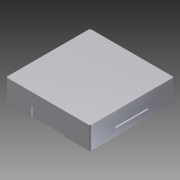
# Autodesk Inventor part: YB16SKW01-05-BB-BBni_lens
Saved by Autodesk Inventor 2014 (Build 180170000, 170)
## iProperties
Category: PARTsolutions
Company: NKKSWITCHES
Created: 2013-12-31
Part Number: YB16SKW01-05-BB-BBni_lens
Catalog Web Link: www.cadenas.de
Description: Panel Mount Non-Illuminated Pushbuttons_ni_lens-
Vendor: NKKSWITCHES
Document SubType Name: Modeling
Designer: PARTuser1
Manufacturer: NKKSWITCHES
Density: 1 g/cm^3
Material: Generic
Appearance: RGB(255.00000000000000,255.00000000000000,255.00000000000000)
PSOL_IDENT_0: {$CADENAS_DATA\23d-libs\nkkswitches\pushbuttons\yb\parts\yb_ni_lens.prj},283 {VTYP=3D},{NB=YB16SKW01
PSOL_IDENT_1: -05-BB-BBni_lens},{LINA=YB16SKW01-05-BB-BBni_lens},{NN=Panel Mount Non-Illuminated Pushbuttons_ni_le
PSOL_IDENT_2: ns},{DATE=23.07.2008 06:28:57},{GEOMDATE=23.07.2008 06:28:00},{VERSION=},{LINEID=10},{LINESUBID=-1},
PSOL_IDENT_3: {WBVAR=PLS,CRCTS,PS,SHPS,CMR,TRMNLS,LMPS,RSSTR,CTCLR,CCLR}  {NB=YB16SKW01-05-BB-BBni_lens},{LINA=YB1
PSOL_IDENT_4: 6SKW01-05-BB-BBni_lens},{KT=DUMMY},{PN=YB16SKW01-05-BB-BB},{SRS=YB},{PLS=1},{CRCTS=6},{PS=},{SHPS=S}
PSOL_IDENT_5: ,{SHPSALG= 'S', 'S - Square (Bushing Mounting)', 'C'  , 'C - Round (Bushing Mounting)', 'R', 'R - Re
PSOL_IDENT_6: ctangular (Bushing Mounting)'  , 'K', 'K - Square (Snap-in Mounting)', 'M', 'M - Round (Snap-in Moun
PSOL_IDENT_7: ting)'  , 'N', 'N - Rectangular (Snap-in Mounting)' },{HSNG=K - Black only},{CMR=W},{TRMNLS=01},{A=0
PSOL_IDENT_8: .709},{A1=0.591},{A11=0.827},{B=0.709},{B1=0.591},{L=0.669},{L1=0.327},{L2=0.957},{L3=0.429},{L4=0.3
PSOL_IDENT_9: 70},{L5=0.118},{L6=0.209},{L7=0.157},{L8=0.480},{DIA1=0.591},{DIA=0.709},{LMPS=05},{LMPS1= '05','05
PSOL_IDENT_10: - 5-volt (Incandescent Lamp used with Solid Cap)', '12','12 - 12-volt (Incandescent Lamp used with S
PSOL_IDENT_11: olid Cap)', '01','01 - 110-volt (Neon used w/ Insert Cap)', '05','05 - 5-volt (Incandescent used w/
PSOL_IDENT_12: Insert Cap)', '12','12 - 12-volt (Incandescent used w/ Insert Cap)', '5C','5C - Red (Bright LED used
PSOL_IDENT_13: with LED Cap)', '5D','5D - Amber (Bright LED used with LED Cap)', '5F','5F - Green (Bright LED used
PSOL_IDENT_14: with LED Cap)', '6B','6B - White (Super Bright LED used with LED Cap)', '6F','6F - Green (Super Bri
PSOL_IDENT_15: ght LED used with LED Cap)', '6G','6G - Blue (Super Bright LED used with LED Cap)', '1C','1C - Red S
PSOL_IDENT_16: ingle Color (LED in Spot Illuminated Cap)', '1D','1D - Amber Single Color (LED in Spot Illuminated C
PSOL_IDENT_17: ap)', '1F','1F - Green Single Color (LED in Spot Illuminated Cap)', 'CF','CF - Red/Green Bicolor (LE
PSOL_IDENT_18: D in Spot Illuminated Cap)' },{RSSTR=},{RSSTR1= '','N/A' },{CTCLR=BB},{CTCLR1= 'BB','BB - White/Whit
PSOL_IDENT_19: e (Solid Cap: Lens/Insert Colors)', 'CB','CB - Red/White (Solid Cap: Lens/Insert Colors)', 'EB','EB
PSOL_IDENT_20: - Yellow/White (Solid Cap: Lens/Insert Colors)', 'FB','FB - Green/White (Solid Cap: Lens/Insert Colo
PSOL_IDENT_21: rs)', 'GB','GB - Blue/White (Solid Cap: Lens/Insert Colors)' },{COLTRANS=1.00,1.00,1.00,0.00},{OCHR=
PSOL_IDENT_22: Download pdf},{NDM=16.000},{COL=1.00,1.00,1.00,0.00},{CCLR=BB}
CNS_NN: Panel Mount Non-Illuminated Pushbuttons_ni_lens
CNS_NB: YB16SKW01-05-BB-BBni_lens
CNS_NBSYN: $PN.ni_lens
CNS_LINA: YB16SKW01-05-BB-BBni_lens
CNS_PN: YB16SKW01-05-BB-BB
CNS_SRS: YB
CNS_PLS: 1 - SPDT
CNS_CRCTS: 6 - ON/ON
CNS_PS: Without Panel Seal
CNS_SHPS: S - Square (Bushing Mounting)
CNS_SHPSALG: 'S', 'S - Square (Bushing Mounting)', 'C'  , 'C - Round (Bushing Mounting)', 'R', 'R - Rectangular (Bushing Mounting)'  , 'K', 'K - Square (Snap-in Mounting)', 'M', 'M - Round (Snap-in Mounting)'  , 'N', 'N - Rectangular (Snap-in Mounting)'
CNS_HSNG: K - Black only
CNS_CMR: W - Silver; Rated 3A @ 125V AC
CNS_TRMNLS: 01 - Solder Lug/.110" (2.8mm) Quick Connect
CNS_A: 0.709
CNS_A1: 0.591
CNS_A11: 0.827
CNS_B: 0.709
CNS_B1: 0.591
CNS_L: 0.669
CNS_L1: 0.327
CNS_L2: 0.957
CNS_L3: 0.429
CNS_L4: 0.370
CNS_L5: 0.118
CNS_L6: 0.209
CNS_L7: 0.157
CNS_L8: 0.480
CNS_DIA1: 0.591
CNS_DIA: 0.709
CNS_LMPS: 05 - 5-volt (Incandescent Lamp for Solid Cap)
CNS_LMPS1: '05','05 - 5-volt (Incandescent Lamp used with Solid Cap)', '12','12 - 12-volt (Incandescent Lamp used with Solid Cap)', '01','01 - 110-volt (Neon used w/ Insert Cap)', '05','05 - 5-volt (Incandescent used w/ Insert Cap)', '12','12 - 12-volt (Incandescent used w/ Insert Cap)', '5C','5C - Red (Bright LED used with LED Cap)', '5D','5D - Amber (Bright LED used with LED Cap)', '5F','5F - Green (Bright LED used with LED Cap)', '6B','6B - White (Super Bright LED used with LED Cap)', '6F','6F - Green (Super Bright LED used with LED Cap)', '6G','6G - Blue (Super Bright LED used with LED Cap)', '1C','1C - Red Single Color (LED in Spot Illuminated Cap)', '1D','1D - Amber Single Color (LED in Spot Illuminated Cap)', '1F','1F - Green Single Color (LED in Spot Illuminated Cap)', 'CF','CF - Red/Green Bicolor (LED in Spot Illuminated Cap)'
CNS_RSSTR: N/A
CNS_RSSTR1: '','N/A'
CNS_CTCLR: BB - White/White (Solid Cap: Lens/Insert Colors)
CNS_CTCLR1: 'BB','BB - White/White (Solid Cap: Lens/Insert Colors)', 'CB','CB - Red/White (Solid Cap: Lens/Insert Colors)', 'EB','EB - Yellow/White (Solid Cap: Lens/Insert Colors)', 'FB','FB - Green/White (Solid Cap: Lens/Insert Colors)', 'GB','GB - Blue/White (Solid Cap: Lens/Insert Colors)'
CNS_COLTRANS: 1.00,1.00,1.00,0.00
CNS_OCHR: Download pdf
CNS_NDM: 16.000
CNS_COL: 1.00,1.00,1.00,0.00
CNS_CCLR: BB - White/White
SUPPLIER: NKKSWITCHES
ARTICLENO: YB16SKW01-05-BB-BBni_lens
BOMINFO: YB16SKW01-05-BB-BBni_lens
CREATOR: CADENAS GmbH
Title: YB16SKW01-05-BB-BBni_lens
Author: Cadenas PARTsolutions
Autodesk Inventor part; units mm, degrees
sketch "Sketch_31" plane through (0, 0, 0) normal (0, 0, 1) x (1, 0, 0)
  line L0 (-7.5057, 3.9878) -> (-7.5057, 0)
  line L1 (-7.5057, 0) -> (7.5057, 0)
  line L2 (7.5057, 0) -> (7.5057, 3.9878)
  line L3 (7.5057, 3.9878) -> (-7.5057, 3.9878)
  constraints: 8 end point
extrude "Extrusion1" add sketch "Sketch_31" along normal mid plane 15.0114
sketch "Sketch_4" plane through (0, 0, 0) normal (0, 0, 1) x (1, 0, 0)
  line L0 (-7.5057, 1.27) -> (-7.2517, 1.27)
  line L1 (-7.2517, 1.27) -> (-7.2517, 1.8682)
  line L2 (-7.2517, 1.8682) -> (-7.5057, 1.8682)
  line L3 (-7.5057, 1.8682) -> (-7.5057, 1.27)
  constraints: 8 end point
extrude "Extrusion2" cut sketch "Sketch_4" along normal mid plane 6.0046
sketch "Sketch_5" plane through (0, 0, 0) normal (0, 0, 1) x (1, 0, 0)
  line L0 (7.2517, 1.27) -> (7.5057, 1.27)
  line L1 (7.5057, 1.27) -> (7.5057, 1.8682)
  line L2 (7.5057, 1.8682) -> (7.2517, 1.8682)
  line L3 (7.2517, 1.8682) -> (7.2517, 1.27)
  constraints: 8 end point
extrude "Extrusion3" cut sketch "Sketch_5" along normal mid plane 6.0046
sketch "Sketch_14" plane through (0, 0, 0) normal (1, 0, 0) x (0, 1, 0)
  line L0 (0, 7.5057) -> (0, 7.2517)
  line L1 (0, 7.2517) -> (1.8682, 7.2517)
  line L2 (1.8682, 7.2517) -> (1.8682, 7.5057)
  line L3 (1.8682, 7.5057) -> (0, 7.5057)
  constraints: 8 end point
extrude "Extrusion4" cut sketch "Sketch_14" along normal mid plane 6.0046
sketch "Sketch_15" plane through (0, 0, 0) normal (1, 0, 0) x (0, 1, 0)
  line L0 (0, -7.2517) -> (0, -7.5057)
  line L1 (0, -7.5057) -> (1.8682, -7.5057)
  line L2 (1.8682, -7.5057) -> (1.8682, -7.2517)
  line L3 (1.8682, -7.2517) -> (0, -7.2517)
  constraints: 8 end point
extrude "Extrusion5" cut sketch "Sketch_15" along normal mid plane 6.0046
sketch "Sketch_8" plane through (0, 0, 0) normal (0, 1, 0) x (-1, 0, 0)
  line L0 (8.2563, 8.2563) -> (-8.2563, 8.2563)
  line L1 (-8.2563, 8.2563) -> (-8.2563, -8.2563)
  line L2 (-8.2563, -8.2563) -> (8.2563, -8.2563)
  line L3 (8.2563, -8.2563) -> (8.2563, 8.2563)
  line L4 (7.5057, -7.2517) -> (7.5057, 7.2517)
  arc A0 (7.5057, 7.2517) -> (7.2517, 7.5057) centre (7.2517, 7.2517) ccw
  line L5 (7.2517, 7.5057) -> (-7.2517, 7.5057)
  arc A1 (-7.2517, 7.5057) -> (-7.5057, 7.2517) centre (-7.2517, 7.2517) ccw
  line L6 (-7.5057, 7.2517) -> (-7.5057, -7.2517)
  arc A2 (-7.5057, -7.2517) -> (-7.2517, -7.5057) centre (-7.2517, -7.2517) ccw
  line L7 (-7.2517, -7.5057) -> (7.2517, -7.5057)
  arc A3 (7.2517, -7.5057) -> (7.5057, -7.2517) centre (7.2517, -7.2517) ccw
  constraints: 16 end point, 8 point on circle, 4 centre point
extrude "Extrusion6" cut sketch "Sketch_8" along normal mid plane 10.5156
ref_plane "lens_to_bicol_led_1_XY" through (1.251, 3.9878, 4.9276) normal (0, 1, 0) x (1, 0, 0)
ref_plane "lens_to_bicol_led_1_YZ" through (1.251, 3.9878, 4.9276) normal (1, 0, 0) x (0, 0, -1)
ref_plane "lens_to_bicol_led_1_ZX" through (1.251, 3.9878, 4.9276) normal (0, 0, -1) x (0, 1, 0)
ref_plane "lens_to_bicol_led_2_XY" through (-1.251, 3.9878, 4.9276) normal (0, 1, 0) x (1, 0, 0)
ref_plane "lens_to_bicol_led_2_YZ" through (-1.251, 3.9878, 4.9276) normal (1, 0, 0) x (0, 0, -1)
ref_plane "lens_to_bicol_led_2_ZX" through (-1.251, 3.9878, 4.9276) normal (0, 0, -1) x (0, 1, 0)
ref_plane "lens_to_insert_XY" through (0, 2.9718, 0) normal (0, 1, 0) x (1, 0, 0)
ref_plane "lens_to_insert_YZ" through (0, 2.9718, 0) normal (1, 0, 0) x (0, 0, -1)
ref_plane "lens_to_insert_ZX" through (0, 2.9718, 0) normal (0, 0, -1) x (0, 1, 0)
ref_plane "lens_to_led_XY" through (0, 3.9878, 4.9276) normal (0, 1, 0) x (1, 0, 0)
ref_plane "lens_to_led_YZ" through (0, 3.9878, 4.9276) normal (1, 0, 0) x (0, 0, -1)
ref_plane "lens_to_led_ZX" through (0, 3.9878, 4.9276) normal (0, 0, -1) x (0, 1, 0)
ref_plane "lens_to_body_XY" through (0, 0, 0) normal (0, 1, 0) x (1, 0, 0)
ref_plane "lens_to_body_YZ" through (0, 0, 0) normal (1, 0, 0) x (0, 0, -1)
ref_plane "lens_to_body_ZX" through (0, 0, 0) normal (0, 0, -1) x (0, 1, 0)
body "Solid1"
